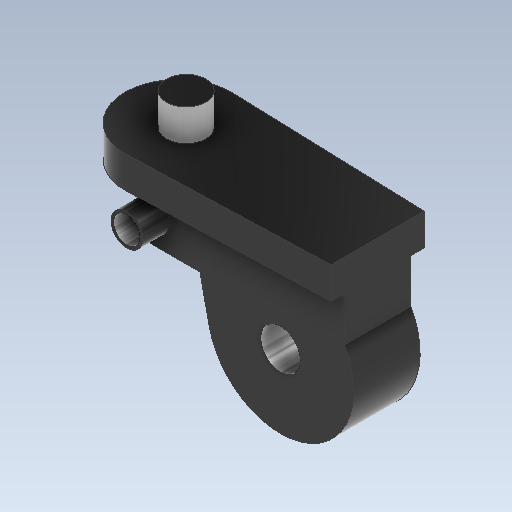
# Autodesk Inventor part: Bracket
Saved by Autodesk Inventor 2021 (Build 250183000, 183)
## iProperties
Created: 2020-07-20
Part Number: Bracket
Material: Generic
Document SubType Name: Modeling
Designer: brook
Density: 1 g/cm^3
Appearance: Default
Mass: 124.351 g
Surface Area: 216.899 cm^2
Volume: 124.351 cm^3
Author: brook
Autodesk Inventor part; units mm, degrees
ref_plane "YZ Plane" through (0, 0, 0) normal (1, 0, 0) x (0, 1, 0)
ref_plane "XZ Plane" through (0, 0, 0) normal (0, 1, 0) x (-1, 0, 0)
ref_plane "XY Plane" through (0, 0, 0) normal (0, 0, 1) x (1, 0, 0)
sketch "Sketch1" plane through (0, 0, 0) normal (0, 1, 0) x (-1, 0, 0)
  arc A0 (-0.6693, -19.9888) -> (-0.6693, 19.9888) centre (0, 0) ccw
  line L0 (-0.6693, 19.9888) -> (-75, 17.5)
  line L1 (-75, 17.5) -> (-75, -17.5)
  line L2 (-75, -17.5) -> (-0.6693, -19.9888)
  dimension "d0" = 40
  dimension "d1" = 75
  dimension "d2" = 35
  dimension "d3" = 17.5
  constraints: 6 end point, 2 point on circle, 2 tangent, 1 centre point, 1 coincident, 1 vertical
  measures "d0" diameter of A0
  measures "d1" distance from line of L1 point (0, 0)
  measures "d2" distance of L0.end L1.end
  measures "d3" vertical distance of point (0, 0) L1.end
extrude "Extrusion1" add sketch "Sketch1" along normal blind 12
sketch "Sketch2" plane through (0, 12, 0) normal (0, 1, 0) x (1, 0, 0)
  circle A0 centre (3, 0) radius 7.5
  point P0 (0, 0)
  dimension "d6" = 15
  dimension "d7" = 0
  dimension "d8" = 3
  constraints: 1 centre point
  measures "d6" diameter of A0
  measures "d7" vertical distance of point (0, 0) A0.centre
  measures "d8" distance of A0.centre point (0, 0)
extrude "Extrusion2" add sketch "Sketch2" along normal blind 12
sketch "Sketch3" plane through (0, 0, 0) normal (0, 0, 1) x (1, 0, 0)
  line L0 (0.6693, 0) -> (-20, 0) projected
  line L1 (-9.3307, 0) -> (-9.3307, -20)
  line L2 (-9.3307, -20) -> (20.6693, -20)
  line L3 (20.6693, -20) -> (24.1328, -35.8653)
  arc A0 (24.1328, -35.8653) -> (75, -16.5743) centre (51, -30) ccw
  line L4 (0.6693, 0) -> (75, 0) projected
  line L5 (75, 0) -> (75, -16.5743)
  line L6 (0.6693, 0) -> (0.6693, 12) projected
  line L7 (75, 0) -> (75, 12) projected
  point P0 (0, 0)
  dimension "d11" = 55
  dimension "d12" = 30
  dimension "d13" = 10
  dimension "d14" = 24
  dimension "d15" = 30
  dimension "d16" = 20
  constraints: 8 end point, 2 point on circle, 2 vertical, 1 centre point, 1 perpendicular, 1 point on line, 1 tangent
  measures "d11" diameter of A0
  measures "d12" distance of L1.end L2.end
  measures "d13" distance between parallel lines of L6 L1
  measures "d14" distance from line of L7 A0.centre
  measures "d15" distance from line of L4 A0.centre
  measures "d16" distance of L1.start L1.end
extrude "Extrusion3" add sketch "Sketch3" along normal mid plane 25
fillet "Fillet1" radius 12.5 2 edges at (-9.3307, -10, 12.5) (-9.3307, -10, -12.5)
sketch "Sketch4" plane through (0, 0, 12.5) normal (0, 0, 1) x (1, 0, 0)
  circle A0 centre (3.1693, -10) radius 5
  line L0 (3.1693, -20) -> (20.6693, -20) projected
  line L1 (3.1693, -20) -> (3.1693, 0) projected
  circle A1 centre (3.1693, -10) radius 6
  point P0 (0, 0)
  dimension "d20" = 10
  dimension "d21" = 10
  dimension "d22" = 0
  dimension "d23" = 12
  constraints: 2 centre point, 1 coincident
  measures "d20" diameter of A0
  measures "d21" distance from line of L0 A0.centre
  measures "d22" distance from line of L1 A0.centre
  measures "d23" diameter of A1
extrude "Extrusion4" add sketch "Sketch4" along normal blind 10 contours A0 L1 A1 | A0 L1 A1
mirror "Mirror1" about plane through (0, 0, 0) normal (0, 0, 1) of "Extrusion4"
sketch "Sketch5" plane through (0, 0, -12.5) normal (0, 0, -1) x (-1, 0, 0)
  circle A0 centre (-51, -30) radius 7.5
  arc A1 (-75, -16.5743) -> (-24.1328, -35.8653) centre (-51, -30) ccw projected
  point P0 (0, 0)
  dimension "d26" = 15
  constraints: 1 centre point, 1 concentric
  measures "d26" diameter of A0
extrude "Extrusion5" cut sketch "Sketch5" against normal through all
body "Solid1"
